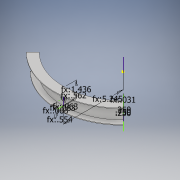
# Autodesk Inventor part: Layer2_Prep
Saved by Autodesk Inventor 2017 (Build 210142000, 142)
## iProperties
Created: 2017-01-26
Part Number: Layer2_Prep
Material: Generic
Document SubType Name: Modeling
Designer: David Kopala
Density: 1 g/cm^3
Appearance: Default
Lay2Rad: 5.245 in
Author: David Kopala
Autodesk Inventor part; units mm, degrees
ref_plane "YZ Plane" through (0, 0, 0) normal (1, 0, 0) x (0, 1, 0)
ref_plane "XZ Plane" through (0, 0, 0) normal (0, 1, 0) x (-1, 0, 0)
ref_plane "XY Plane" through (0, 0, 0) normal (0, 0, 1) x (1, 0, 0)
sketch "Sketch1" plane through (0, 0, 0) normal (1, 0, 0) x (0, 1, 0)
  line L0 (0, 0) -> (28.6807, 0)
  line L1 (0, 133.2109) -> (36.4852, 133.2109)
  line L2 (0, 133.2109) -> (0, 147.2732)
  line L3 (0, 147.2732) -> (1.5875, 147.2732)
  line L4 (1.5875, 134.7984) -> (36.4852, 134.7984)
  line L5 (36.4852, 134.7984) -> (36.4852, 133.2109)
  line L6 (1.5875, 134.7984) -> (1.5875, 147.2732)
  point P0 (15.8613, 134.7984)
  dimension "Lay2Rad" = 133.2109
  dimension "d1" = 14.0623
  dimension "d2" = 1.5875
  dimension "d3" = 36.4852
  dimension "d4" = 1.5875
  dimension "d5" = 1.5875
  dimension "d7" = 14.2738
  constraints: 14 end point, 4 horizontal, 1 perpendicular, 1 point on line, 1 vertical
  measures "Lay2Rad" distance between parallel lines of L0 L1
  measures "d1" distance of L1.start L2.end
  measures "d2" distance of L2.end L3.end
  measures "d3" distance of L1.start L1.end
  measures "d4" distance from line of L2 L4.start
  measures "d5" distance from line of L1 L4.start
  measures "d7" distance from line of L6 point (15.861, 134.798)
revolve "Revolution1" add sketch "Sketch1" angle 360 about axis through (0, 0, 0) along (0, 1, 0)
ref_plane "Work Plane1" through (0, 15.8613, 134.7984) normal (0, 0, 1) x (1, 0, 0)
sketch "Sketch2" plane through (0, 15.8613, 134.7984) normal (0, 0, 1) x (1, 0, 0)
  circle A0 centre (0, 0) radius 4.7625
  circle A1 centre (0, 0) radius 3.9688
  point P0 (0, -15.8613)
  dimension "d8" = 9.525
  dimension "d11" = 7.9375
  constraints: 2 centre point, 1 coincident
  measures "d8" diameter of A0
  measures "d11" diameter of A1
extrude "Extrusion2" cut sketch "Sketch2" against normal through all contours A1
extrude "Extrusion3" add sketch "Sketch2" along normal blind 0.3969
sketch "Sketch3" plane through (0, 36.4852, 0) normal (0, 1, 0) x (1, 0, 0)
  circle A0 centre (0, 0) radius 133.2109
  circle A1 centre (0, 0) radius 133.2109 projected
  circle A2 centre (0, 0) radius 153.6232
  circle A3 centre (0, 0) radius 147.2732 projected
  dimension "d16" = 6.35
  constraints: 2 centre point, 2 coincident, 1 concentric
  measures "d16" radial gap between concentric circles of A3 A2
extrude "Extrusion4" add sketch "Sketch3" along normal blind 1.5875 contours A2 | A3
sketch "Sketch4" plane through (0, 38.0727, 0) normal (0, 1, 0) x (1, 0, 0)
  line L0 (0, 0) -> (-167.0067, -167.0067)
  line L1 (0, 0) -> (236.1832, 0) construction
  line L2 (0, 0) -> (195.6261, -195.6261)
  line L3 (195.6261, -195.6261) -> (-166.4474, -166.4474)
  line L4 (-166.4474, -166.4474) -> (-176.2344, 211.1551)
  line L5 (-176.2344, 211.1551) -> (203.4461, 189.6497)
  line L6 (203.4461, 189.6497) -> (195.6261, -195.6261)
  dimension "d19" = 135
  constraints: 14 end point, 1 equal length, 1 horizontal, 1 point on line
  measures "d19" angle of L0 L1
extrude "Extrusion5" cut sketch "Sketch4" against normal through all contours L0 L4 L5 L6 L2
sketch "Sketch5" plane through (94.1943, 0, 94.1943) normal (0.7071068, 0, -0.7071068) x (-0.7071068, 0, -0.7071068)
  line L0 (-6.6801, 19.05) -> (6.1276, 19.05)
  line L1 (0, 0) -> (-14.0623, 0) projected
  line L2 (0, 38.0727) -> (0, 0) projected
  line L3 (-0.7937, 19.05) -> (-0.7937, 25.4)
  line L4 (-0.7937, 25.4) -> (0, 25.4)
  line L5 (-0.7937, 19.05) -> (-0.7937, 12.7)
  line L6 (-0.7937, 12.7) -> (-1.5875, 12.7)
  line L7 (-1.5875, 1.5875) -> (-1.5875, 36.4852) projected
  line L8 (-1.5875, 12.7) -> (-21.1154, 12.7)
  line L9 (-21.1154, 12.7) -> (-9.8215, -14.1735)
  line L10 (-9.8215, -14.1735) -> (10.1035, -9.9498)
  line L11 (10.1035, -9.9498) -> (6.1276, 19.05)
  line L12 (0, 25.4) -> (7.2571, 44.9587)
  line L13 (7.2571, 44.9587) -> (-27.8182, 42.4796)
  line L14 (-27.8182, 42.4796) -> (-19.0035, 23.7483)
  line L15 (-19.0035, 23.7483) -> (-6.3412, 19.05)
  point P0 (133.2109, 0)
  dimension "d22" = 19.05
  dimension "d23" = 0.7937
  dimension "d24" = 6.35
  dimension "d25" = 6.35
  constraints: 26 end point, 5 point on line, 3 perpendicular, 2 horizontal, 1 vertical
  measures "d22" distance between parallel lines of L1 L0
  measures "d23" distance from line of L2 L3.start
  measures "d24" distance of L3.start L3.end
  measures "d25" distance of L3.start L5.end
equation "\"Lay2Rad\" = -2 * SpWall + 0.5 * IBDia"
equation "\"d2\" = Wall"
equation "\"d3\" = d1_1 + BevDriverDia + SpWall + Space + Wall"
equation "\"d4\" = Wall"
equation "\"d5\" = Wall"
equation "\"d7\" = 1.5 * Space + 0.5 * BevDriverDia"
equation "\"d8\" = 2 * Space + AxelDia"
equation "\"d11\" = AxelDia + Space"
equation "\"d14\" = 0.25 * Wall"
equation "\"d17\" = Wall"
equation "\"d23\" = 0.5 * Wall"
equation "\"SpWall\" = 3.175"
equation "\"IBDia\" = 279.121792"
equation "\"Wall\" = 1.5875"
equation "\"d1_1\" = 6.35"
equation "\"BevDriverDia\" = 23.785175"
equation "\"Space\" = 1.5875"
equation "\"AxelDia\" = 6.35"
body "Solid1"
